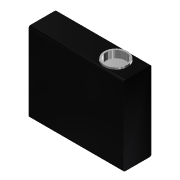
# Autodesk Inventor part: Projector-AcerP1500
Saved by Autodesk Inventor 2014 (Build 180170000, 170)
## iProperties
Created: 2014-08-10
Part Number: Projector-AcerP1500
Material: Generic
Document SubType Name: Modeling
Designer: Peele
Density: 1 g/cm^3
Appearance: Default
Author: Peele
Autodesk Inventor part; units mm, degrees
ref_plane "YZ Plane" through (0, 0, 0) normal (1, 0, 0) x (0, 1, 0)
ref_plane "XZ Plane" through (0, 0, 0) normal (0, 1, 0) x (-1, 0, 0)
ref_plane "XY Plane" through (0, 0, 0) normal (0, 0, 1) x (1, 0, 0)
sketch "Sketch1" plane through (0, 0, 0) normal (0, 1, 0) x (-1, 0, 0)
  line L0 (-132.08, -110.49) -> (132.08, -110.49)
  line L1 (132.08, -110.49) -> (132.08, 110.49)
  line L2 (132.08, 110.49) -> (-132.08, 110.49)
  line L3 (-132.08, 110.49) -> (-132.08, -110.49)
  line L4 (-132.08, -110.49) -> (132.08, 110.49) construction
  line L5 (132.08, -110.49) -> (-132.08, 110.49) construction
  point P0 (0, 0)
  dimension "d0" = 264.16
  dimension "d1" = 220.98
  constraints: 12 end point, 2 midpoint, 2 parallel, 1 horizontal, 1 perpendicular
  measures "d0" distance of L1.end L2.end
  measures "d1" distance of L2.end L0.start
extrude "Extrusion1" add sketch "Sketch1" along normal blind 78.74
sketch "Sketch2" plane through (-132.08, 0, 110.49) normal (0, 0, 1) x (1, 0, 0)
  line L0 (264.16, 0) -> (264.16, 78.74) projected
  line L1 (0, 78.74) -> (264.16, 78.74) projected
  circle A0 centre (204.16, 39.37) radius 32.5
  point P0 (0, 0)
  point P1 (132.08, 0)
  dimension "d4" = 60
  dimension "d5" = 65
  dimension "d6" = 78.74
  dimension "d7" = 39.37
  constraints: 1 centre point
  measures "d4" distance from line of A0.centre L0
  measures "d5" diameter of A0
  measures "d6" distance of point (0, 0) L1.start
  measures "d7" distance from line of A0.centre L1
extrude "Extrusion2" add sketch "Sketch2" along normal blind 5
sketch "Sketch3" plane through (72.08, 39.37, 115.49) normal (0, 0, 1) x (1, 0, 0)
  circle A0 centre (0, 0) radius 32.5 projected
  circle A1 centre (0, 0) radius 27.5
  point P0 (-72.08, -39.37)
  dimension "d10" = 55
  constraints: 1 centre point, 1 coincident
  measures "d10" diameter of A1
extrude "Extrusion3" cut sketch "Sketch3" against normal blind 20 contours A1
fillet "Fillet1" radius 6 4 edges at (0, 78.74, 110.49) (0, 78.74, -110.49) (0, 0, -110.49) (0, 0, 110.49)
fillet "Fillet2" radius 1 16 edges at (-132.08, 76.9826, 108.7326) (-132.08, 78.74, 0) (-132.08, 76.9826, -108.7326) (-132.08, 39.37, -110.49) (-132.08, 1.7574, -108.7326) (-132.08, 0, 0) (-132.08, 1.7574, 108.7326) (-132.08, 39.37, 110.49) (132.08, 76.9826, -108.7326) (132.08, 39.37, -110.49) (132.08, 1.7574, -108.7326) (132.08, 0, 0) (132.08, 1.7574, 108.7326) (132.08, 39.37, 110.49) (132.08, 76.9826, 108.7326) (132.08, 78.74, 0)
equation "\"d7\" = 0.5 * d6"
body "Solid1"
